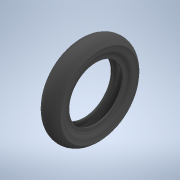
# Autodesk Inventor part: tyre-10x2_125
Saved by Autodesk Inventor 2022 (Build 260153000, 153)
## iProperties
Created: 2025-01-14
Part Number: tyre-10x2_125
Material: Generic
Document SubType Name: Modeling
Designer: Kostic
Density: 1 g/cm^3
Appearance: Default
Author: Kostic
Autodesk Inventor part; units mm, degrees
ref_plane "YZ Plane" through (0, 0, 0) normal (1, 0, 0) x (0, 1, 0)
ref_plane "XZ Plane" through (0, 0, 0) normal (0, 1, 0) x (-1, 0, 0)
ref_plane "XY Plane" through (0, 0, 0) normal (0, 0, 1) x (1, 0, 0)
sketch "Sketch1" plane through (0, 0, 0) normal (0, 0, 1) x (1, 0, 0)
  line L0 (0, 0) -> (17, 0)
  line L1 (17, 0) -> (17, 6)
  line L2 (0, 0) -> (0, 49)
  arc A0 (27.5, 34) -> (0, 49) centre (0, 16.2917) ccw
  arc A1 (19, 12) -> (17, 6) centre (27, 6) ccw
  arc A2 (27.5, 34) -> (24.9341, 22.5257) centre (56.7418, 21.4368) ccw
  arc A3 (19, 12) -> (24.9341, 22.5257) centre (11.8368, 22.974) ccw
  line L3 (0, -76) -> (59.1269, -76)
  dimension "d0" = 17
  dimension "d1" = 6
  dimension "d2" = 49
  dimension "d3" = 34
  dimension "d4" = 27.5
  dimension "d5" = 6
  dimension "d6" = 2
  dimension "d7" = 125
  constraints: 8 end point, 8 point on circle, 4 centre point, 2 horizontal, 2 tangent, 1 line through centre, 1 perpendicular, 1 vertical
  measures "d0" distance of L0.start L0.end
  measures "d1" distance of L0.end L1.end
  measures "d2" distance of L0.start L2.end
  measures "d3" vertical distance of L0.start A0.start
  measures "d4" distance from line of L2 A0.start
  measures "d5" vertical distance of L1.end A1.start
  measures "d6" horizontal distance of L1.end A1.start
  measures "d7" distance from line of L3 L2.end
revolve "Revolution1" add sketch "Sketch1" angle 360 about axis through (0, -76, 0) along (1, 0, 0)
mirror "Mirror1" about plane through (0, 49, 0) normal (-1, 0, 0)
shell "Shell1" thickness 4 removed faces 1 at (5.6667, -120.8366, 61.3651)
body "Solid1"
